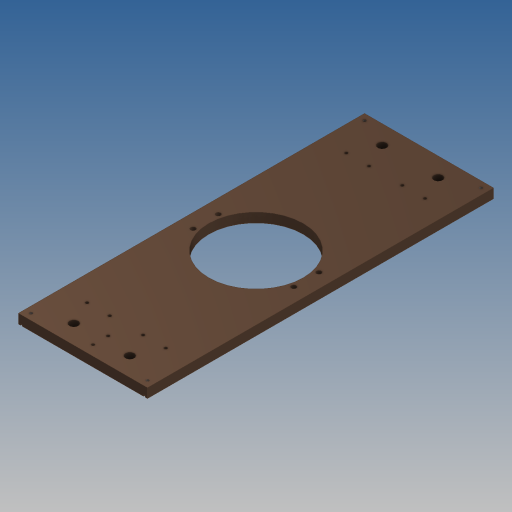
# Autodesk Inventor part: Grundplatte 2.0
Saved by Autodesk Inventor 2023.3 (Build 273359000, 359)
## iProperties
Created: 2021-10-11
Part Number: Grundplatte 2.0
Material: Generisch
Document SubType Name: Modeling
Designer: bhelg
Density: 1 g/cm^3
Appearance: Vorgabe
Author: bhelg
Autodesk Inventor part; units mm, degrees
ref_plane "YZ Plane" through (0, 0, 0) normal (1, 0, 0) x (0, 1, 0)
ref_plane "XZ Plane" through (0, 0, 0) normal (0, 1, 0) x (-1, 0, 0)
ref_plane "XY Plane" through (0, 0, 0) normal (0, 0, 1) x (1, 0, 0)
sketch "Skizze2" plane through (0, 0, 0) normal (0, 1, 0) x (-1, 0, 0)
  circle A0 centre (0, 0) radius 75
  line L0 (-102.5, -275) -> (102.5, -275)
  line L1 (102.5, -275) -> (102.5, 275)
  line L2 (102.5, 275) -> (-102.5, 275)
  line L3 (-102.5, 275) -> (-102.5, -275)
  line L4 (-102.5, -275) -> (102.5, 275) construction
  line L5 (102.5, -275) -> (-102.5, 275) construction
  dimension "d8" = 150
  dimension "d9" = 205
  dimension "d10" = 550
  constraints: 12 end point, 2 midpoint, 2 parallel, 1 centre point, 1 coincident, 1 horizontal, 1 perpendicular
  measures "d8" diameter of A0
  measures "d9" distance of L2.end L1.end
  measures "d10" distance of L1.end L0.end
extrude "Extrusion1" add sketch "Skizze2" along normal blind 15
sketch "Skizze3" plane through (0, 0, 0) normal (0, -1, 0) x (1, 0, 0)
  line L0 (-92.5, -265) -> (92.5, -265)
  line L1 (92.5, -265) -> (92.5, 265)
  line L2 (92.5, 265) -> (-92.5, 265)
  line L3 (-92.5, 265) -> (-92.5, -265)
  line L4 (-92.5, -265) -> (92.5, 265) construction
  line L5 (92.5, -265) -> (-92.5, 265) construction
  line L6 (-102.5, -275) -> (-102.5, 275) projected
  line L7 (102.5, 275) -> (102.5, -275) projected
  point P0 (0, 0)
  dimension "d13" = 185
  dimension "d14" = 530
  dimension "d86" = 205
  constraints: 12 end point, 2 midpoint, 2 parallel, 1 horizontal, 1 perpendicular
  measures "d13" distance of L2.end L1.end
  measures "d14" distance of L1.end L0.end
  measures "d86" distance between parallel lines of L6 L7
hole "Bohrung1" at (92.5, 0, -265) at (-92.5, 0, -265) at (-92.5, 0, 265) at (92.5, 0, 265) direction (0, 1, 0) diameter 4.917 end through all thread size "M6x1" class "6H" standard "ISO Metric profile"
sketch "Skizze6" plane through (0, 0, 0) normal (0, -1, 0) x (1, 0, 0)
  line L0 (99, 275) -> (99, -275)
  line L1 (102.5, 275) -> (102.5, -275) projected
  line L2 (96.5, 275) -> (96.5, -275)
  line L3 (-99, -275) -> (-99, 275)
  line L4 (-96.5, -275) -> (-96.5, 275)
  line L5 (102.5, -275) -> (-102.5, -275) projected
  line L6 (96.5, -275) -> (99, -275)
  line L7 (-96.5, -275) -> (-99, -275)
  line L8 (-102.5, 275) -> (102.5, 275) projected
  line L9 (-96.5, 275) -> (-99, 275)
  line L10 (99, 275) -> (96.5, 275)
  line L11 (-102.5, -275) -> (-102.5, 275) projected
  point P0 (0, 0)
  point P1 (99, 275)
  point P2 (96.5, 275)
  dimension "d68" = 2.5
  dimension "d70" = 2.5
  dimension "d84" = 198
  dimension "d85" = 99
  constraints: 16 end point, 8 point on line, 2 parallel, 2 vertical
  measures "d68" distance between parallel lines of L2 L0
  measures "d70" distance between parallel lines of L3 L4
  measures "d84" distance between parallel lines of L3 L0
  measures "d85" distance from line of point (0, 0) L0
extrude "Extrusion2" cut sketch "Skizze6" against normal blind 2.5 contours L0 L5 L2 L8 | L4 L5 L3 L8
sketch "Skizze7" plane through (0, 0, 0) normal (0, -1, 0) x (1, 0, 0)
  line L0 (-80, -20) -> (80, -20)
  line L1 (80, -20) -> (80, 20)
  line L2 (80, 20) -> (-80, 20)
  line L3 (-80, 20) -> (-80, -20)
  line L4 (-80, -20) -> (80, 20) construction
  line L5 (80, -20) -> (-80, 20) construction
  point P0 (0, 0)
  dimension "d74" = 160
  dimension "d75" = 40
  constraints: 12 end point, 2 midpoint, 2 parallel, 1 horizontal, 1 perpendicular
  measures "d74" distance of L2.end L1.end
  measures "d75" distance of L0.end L1.end
hole "Bohrung6" at (-80, 0, 20) at (-80, 0, -20) at (80, 0, -20) at (80, 0, 20) direction (0, 1, 0) diameter 8 end through all
sketch "Skizze8" plane through (0, 0, 0) normal (0, -1, 0) x (1, 0, 0)
  line L0 (-62.5, -206) -> (62.5, -206)
  line L1 (62.5, -206) -> (62.5, 206)
  line L2 (62.5, 206) -> (-62.5, 206)
  line L3 (-62.5, 206) -> (-62.5, -206)
  line L4 (-62.5, -206) -> (62.5, 206) construction
  line L5 (62.5, -206) -> (-62.5, 206) construction
  line L6 (-26.5, -206) -> (26.5, -206)
  line L7 (26.5, -206) -> (26.5, 206)
  line L8 (26.5, 206) -> (-26.5, 206)
  line L9 (-26.5, 206) -> (-26.5, -206)
  line L10 (-26.5, -206) -> (26.5, 206) construction
  line L11 (26.5, -206) -> (-26.5, 206) construction
  point P0 (0, 0)
  dimension "d87" = 125
  dimension "d88" = 412
  dimension "d89" = 53
  dimension "d90" = 412
  constraints: 24 end point, 4 midpoint, 4 parallel, 2 horizontal, 2 perpendicular
  measures "d87" distance of L2.end L1.end
  measures "d88" distance of L0.end L1.end
  measures "d89" distance of L8.end L7.end
  measures "d90" distance of L7.end L6.end
hole "Bohrung7" at (-62.5, 0, 206) at (-26.5, 0, 206) at (26.5, 0, 206) at (62.5, 0, 206) at (62.5, 0, -206) at (26.5, 0, -206) at (-26.5, 0, -206) at (-62.5, 0, -206) direction (0, 1, 0) diameter 4.917 end through all thread size "M6x1" class "6H" standard "ISO Metric profile"
sketch "Skizze9" plane through (0, 0, 0) normal (0, -1, 0) x (1, 0, 0)
  line L0 (-44.5, -245) -> (44.5, -245)
  line L1 (44.5, -245) -> (44.5, 245)
  line L2 (44.5, 245) -> (-44.5, 245)
  line L3 (-44.5, 245) -> (-44.5, -245)
  line L4 (-44.5, -245) -> (44.5, 245) construction
  line L5 (44.5, -245) -> (-44.5, 245) construction
  line L6 (102.5, 275) -> (102.5, -275) projected
  point P0 (0, 0)
  dimension "d98" = 490
  dimension "d99" = 58
  constraints: 12 end point, 2 midpoint, 2 parallel, 1 horizontal, 1 perpendicular
  measures "d98" distance of L0.end L1.end
  measures "d99" distance between parallel lines of L1 L6
hole "Bohrung8" at (44.5, 0, 245) at (-44.5, 0, 245) at (-44.5, 0, -245) at (44.5, 0, -245) direction (0, 1, 0) diameter 14 end through all
sketch "Skizze10" plane through (0, 0, 0) normal (0, -1, 0) x (1, 0, 0)
  line L0 (-96.5, 275) -> (96.5, 275) projected
  line L1 (-102.5, -275) -> (-102.5, 275) projected
  point P0 (0, 0)
  point P1 (0, 235)
  point P2 (0, 259)
  dimension "d107" = 40
  dimension "d108" = 102.5
  dimension "d116" = 16
  dimension "d117" = 102.5
  measures "d107" distance from line of point (0, 235) L0
  measures "d108" distance from line of L1 point (0, 235)
  measures "d116" distance from line of L0 point (0, 259)
  measures "d117" distance from line of L1 point (0, 259)
hole "Bohrung9" at (0, 0, 235) direction (0, 1, 0) diameter 4.917 end through all thread size "M6x1" class "6H" standard "ISO Metric profile"
sketch "Skizze11" plane through (0, 0, 0) normal (0, -1, 0) x (1, 0, 0)
  line L0 (-102.5, -275) -> (-102.5, 275) projected
  line L1 (-96.5, 275) -> (96.5, 275) projected
  point P0 (0, 0)
  point P1 (0, 259)
  dimension "d118" = 102.5
  dimension "d119" = 16
  measures "d118" distance from line of L0 point (0, 259)
  measures "d119" distance from line of L1 point (0, 259)
hole "Bohrung10" at (0, 0, 259) direction (0, 1, 0) diameter 5 end through all
equation "\"d70\" = d68"
equation "\"d85\" = 0.5 * d84"
